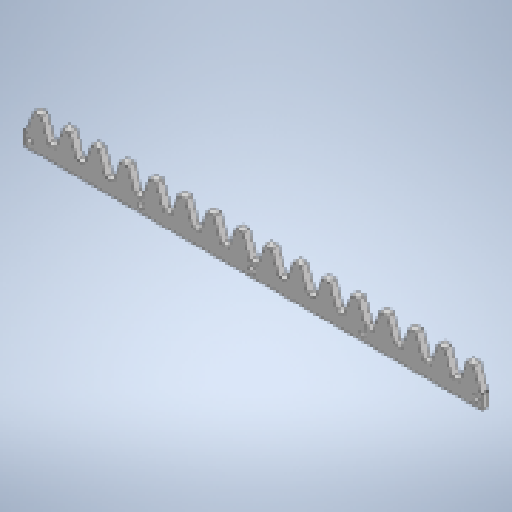
# Autodesk Inventor part: SR4-500_On
Saved by Autodesk Inventor 2024 (Build 280153000, 153)
## iProperties
Created: 2024-06-08
Part Number: SR4-500_On
Material: Generic
Catalog Web Link: www.cadenas.de
Description: Racks (SR)-
Vendor: KHK
Document SubType Name: Modeling
Designer: psAdmin
Manufacturer: KHK
Mass: 817.7 g
Surface Area: 1047.63 cm^2
Volume: 817.7 cm^3
Density: 1 g/cm^3
Appearance: PSOLRGB-175-175-175
Category: PARTsolutions
Company: KHK
PSOL_IDENT_0: {$CADENAS_DATA/23d-libs/khk/racks/racks_sr.prj},167 {VTYP=3D},{NB=SR4-500_On},{LINA=SR4-500},{NN=Rac
PSOL_IDENT_1: ks (SR)},{DATE=12.04.2024 02:30:43},{GEOMDATE=26.02.2019 12:12:45},{VERSION=},{LINEID=330},{WBVAR=TO
PSOL_IDENT_2: OTH},{WBNUMERIC=}  {NB=SR4-500_On},{LINA=SR4-500},{KT=DUMMY},{CN=SR4-500},{M=4.0},{A=505},{B=40},{C=
PSOL_IDENT_3: 45.0},{D=41.0},{ENT=39},{S=R1},{WMF=r1004},{TOOTH=On}
NB: SR4-500_On
NN: Racks (SR)
NBSYN: $CN._$TOOTH.
LINA: SR4-500
CATALOG: KHK
CN: SR4-500
M: 4
A: 505
B: 40
C: 45
D: 41
ENT: 39
S: R1
TOOTH: On
SUPPLIER: KHK
ARTICLENO: SR4-500_On
BOMINFO: SR4-500
CREATOR: CADENAS GmbH
Title: SR4-500
Author: Cadenas PARTsolutions
Autodesk Inventor part; units mm, degrees
ref_plane "YZ Plane" through (0, 0, 0) normal (1, 0, 0) x (0, 1, 0)
ref_plane "XZ Plane" through (0, 0, 0) normal (0, 1, 0) x (-1, 0, 0)
ref_plane "XY Plane" through (0, 0, 0) normal (0, 0, 1) x (1, 0, 0)
sketch "Sketch_4" plane through (0, 0, 0) normal (0, 0, 1) x (1, 0, 0)
  line L0 (0, 45) -> (0, 0)
  line L1 (0, 0) -> (505, 0)
  line L2 (505, 0) -> (505, 45)
  line L3 (505, 45) -> (0, 45)
  constraints: 8 end point
extrude "Extrusion1" add sketch "Sketch_4" along normal mid plane 40
sketch "Sketch_5" plane through (0, 0, 0) normal (0, 0, 1) x (1, 0, 0)
  line L0 (-4.714, 45) -> (-1.57, 36)
  line L1 (-1.57, 36) -> (1.57, 36)
  line L2 (1.57, 36) -> (4.714, 45)
  line L3 (4.714, 45) -> (-4.714, 45)
  constraints: 8 end point
extrude "Extrusion2" cut sketch "Sketch_5" along normal mid plane 40
pattern_linear "Rectangular Pattern1" count 42 spacing 12.56636 along (1, 0, 0) of "Extrusion2"
sketch "スケッチ3" plane through (0, 0, 20) normal (0, 0, 1) x (1, 0, 0)
  line L0 (505, 38.220229) -> (504.2244, 36)
  line L1 (504.2244, 36) -> (501.0844, 36)
  line L2 (501.0844, 36) -> (497.9404, 45)
  line L3 (497.9404, 45) -> (494.80204, 45)
  line L4 (494.80204, 45) -> (491.65804, 36)
  line L5 (491.65804, 36) -> (488.51804, 36)
  line L6 (488.51804, 36) -> (485.37404, 45)
  line L7 (485.37404, 45) -> (482.23568, 45)
  line L8 (482.23568, 45) -> (479.09168, 36)
  line L9 (479.09168, 36) -> (475.95168, 36)
  line L10 (475.95168, 36) -> (472.80768, 45)
  line L11 (472.80768, 45) -> (469.66932, 45)
  line L12 (469.66932, 45) -> (466.52532, 36)
  line L13 (466.52532, 36) -> (463.38532, 36)
  line L14 (463.38532, 36) -> (460.24132, 45)
  line L15 (460.24132, 45) -> (457.10296, 45)
  line L16 (457.10296, 45) -> (453.95896, 36)
  line L17 (453.95896, 36) -> (450.81896, 36)
  line L18 (450.81896, 36) -> (447.67496, 45)
  line L19 (447.67496, 45) -> (444.5366, 45)
  line L20 (444.5366, 45) -> (441.3926, 36)
  line L21 (441.3926, 36) -> (438.2526, 36)
  line L22 (438.2526, 36) -> (435.1086, 45)
  line L23 (435.1086, 45) -> (431.97024, 45)
  line L24 (431.97024, 45) -> (428.82624, 36)
  line L25 (428.82624, 36) -> (425.68624, 36)
  line L26 (425.68624, 36) -> (422.54224, 45)
  line L27 (422.54224, 45) -> (419.40388, 45)
  line L28 (419.40388, 45) -> (416.25988, 36)
  line L29 (416.25988, 36) -> (413.11988, 36)
  line L30 (413.11988, 36) -> (409.97588, 45)
  line L31 (409.97588, 45) -> (406.83752, 45)
  line L32 (406.83752, 45) -> (403.69352, 36)
  line L33 (403.69352, 36) -> (400.55352, 36)
  line L34 (400.55352, 36) -> (397.40952, 45)
  line L35 (397.40952, 45) -> (394.27116, 45)
  line L36 (394.27116, 45) -> (391.12716, 36)
  line L37 (391.12716, 36) -> (387.98716, 36)
  line L38 (387.98716, 36) -> (384.84316, 45)
  line L39 (384.84316, 45) -> (381.7048, 45)
  line L40 (381.7048, 45) -> (378.5608, 36)
  line L41 (378.5608, 36) -> (375.4208, 36)
  line L42 (375.4208, 36) -> (372.2768, 45)
  line L43 (372.2768, 45) -> (369.13844, 45)
  line L44 (369.13844, 45) -> (365.99444, 36)
  line L45 (365.99444, 36) -> (362.85444, 36)
  line L46 (362.85444, 36) -> (359.71044, 45)
  line L47 (359.71044, 45) -> (356.57208, 45)
  line L48 (356.57208, 45) -> (353.42808, 36)
  line L49 (353.42808, 36) -> (350.28808, 36)
  line L50 (350.28808, 36) -> (347.14408, 45)
  line L51 (347.14408, 45) -> (344.00572, 45)
  line L52 (344.00572, 45) -> (340.86172, 36)
  line L53 (340.86172, 36) -> (337.72172, 36)
  line L54 (337.72172, 36) -> (334.57772, 45)
  line L55 (334.57772, 45) -> (331.43936, 45)
  line L56 (331.43936, 45) -> (328.29536, 36)
  line L57 (328.29536, 36) -> (325.15536, 36)
  line L58 (325.15536, 36) -> (322.01136, 45)
  line L59 (322.01136, 45) -> (318.873, 45)
  line L60 (318.873, 45) -> (315.729, 36)
  line L61 (315.729, 36) -> (312.589, 36)
  line L62 (312.589, 36) -> (309.445, 45)
  line L63 (309.445, 45) -> (306.30664, 45)
  line L64 (306.30664, 45) -> (303.16264, 36)
  line L65 (303.16264, 36) -> (300.02264, 36)
  line L66 (300.02264, 36) -> (296.87864, 45)
  line L67 (296.87864, 45) -> (293.74028, 45)
  line L68 (293.74028, 45) -> (290.59628, 36)
  line L69 (290.59628, 36) -> (287.45628, 36)
  line L70 (287.45628, 36) -> (284.31228, 45)
  line L71 (284.31228, 45) -> (281.17392, 45)
  line L72 (281.17392, 45) -> (278.02992, 36)
  line L73 (278.02992, 36) -> (274.88992, 36)
  line L74 (274.88992, 36) -> (271.74592, 45)
  line L75 (271.74592, 45) -> (268.60756, 45)
  line L76 (268.60756, 45) -> (265.46356, 36)
  line L77 (265.46356, 36) -> (262.32356, 36)
  line L78 (262.32356, 36) -> (259.17956, 45)
  line L79 (259.17956, 45) -> (256.0412, 45)
  line L80 (256.0412, 45) -> (252.8972, 36)
  line L81 (252.8972, 36) -> (249.7572, 36)
  line L82 (249.7572, 36) -> (246.6132, 45)
  line L83 (246.6132, 45) -> (243.47484, 45)
  line L84 (243.47484, 45) -> (240.33084, 36)
  line L85 (240.33084, 36) -> (237.19084, 36)
  line L86 (237.19084, 36) -> (234.04684, 45)
  line L87 (234.04684, 45) -> (230.90848, 45)
  line L88 (230.90848, 45) -> (227.76448, 36)
  line L89 (227.76448, 36) -> (224.62448, 36)
  line L90 (224.62448, 36) -> (221.48048, 45)
  line L91 (221.48048, 45) -> (218.34212, 45)
  line L92 (218.34212, 45) -> (215.19812, 36)
  line L93 (215.19812, 36) -> (212.05812, 36)
  line L94 (212.05812, 36) -> (208.91412, 45)
  line L95 (208.91412, 45) -> (205.77576, 45)
  line L96 (205.77576, 45) -> (202.63176, 36)
  line L97 (202.63176, 36) -> (199.49176, 36)
  line L98 (199.49176, 36) -> (196.34776, 45)
  line L99 (196.34776, 45) -> (193.2094, 45)
  line L100 (193.2094, 45) -> (190.0654, 36)
  line L101 (190.0654, 36) -> (186.9254, 36)
  line L102 (186.9254, 36) -> (183.7814, 45)
  line L103 (183.7814, 45) -> (180.64304, 45)
  line L104 (180.64304, 45) -> (177.49904, 36)
  line L105 (177.49904, 36) -> (174.35904, 36)
  line L106 (174.35904, 36) -> (171.21504, 45)
  line L107 (171.21504, 45) -> (168.07668, 45)
  line L108 (168.07668, 45) -> (164.93268, 36)
  line L109 (164.93268, 36) -> (161.79268, 36)
  line L110 (161.79268, 36) -> (158.64868, 45)
  line L111 (158.64868, 45) -> (155.51032, 45)
  line L112 (155.51032, 45) -> (152.36632, 36)
  line L113 (152.36632, 36) -> (149.22632, 36)
  line L114 (149.22632, 36) -> (146.08232, 45)
  line L115 (146.08232, 45) -> (142.94396, 45)
  line L116 (142.94396, 45) -> (139.79996, 36)
  line L117 (139.79996, 36) -> (136.65996, 36)
  line L118 (136.65996, 36) -> (133.51596, 45)
  line L119 (133.51596, 45) -> (130.3776, 45)
  line L120 (130.3776, 45) -> (127.2336, 36)
  line L121 (127.2336, 36) -> (124.0936, 36)
  line L122 (124.0936, 36) -> (120.9496, 45)
  line L123 (120.9496, 45) -> (117.81124, 45)
  line L124 (117.81124, 45) -> (114.66724, 36)
  line L125 (114.66724, 36) -> (111.52724, 36)
  line L126 (111.52724, 36) -> (108.38324, 45)
  line L127 (108.38324, 45) -> (105.24488, 45)
  line L128 (105.24488, 45) -> (102.10088, 36)
  line L129 (102.10088, 36) -> (98.96088, 36)
  line L130 (98.96088, 36) -> (95.81688, 45)
  line L131 (95.81688, 45) -> (92.67852, 45)
  line L132 (92.67852, 45) -> (89.53452, 36)
  line L133 (89.53452, 36) -> (86.39452, 36)
  line L134 (86.39452, 36) -> (83.25052, 45)
  line L135 (83.25052, 45) -> (80.11216, 45)
  line L136 (80.11216, 45) -> (76.96816, 36)
  line L137 (76.96816, 36) -> (73.82816, 36)
  line L138 (73.82816, 36) -> (70.68416, 45)
  line L139 (70.68416, 45) -> (67.5458, 45)
  line L140 (67.5458, 45) -> (64.4018, 36)
  line L141 (64.4018, 36) -> (61.2618, 36)
  line L142 (61.2618, 36) -> (58.1178, 45)
  line L143 (58.1178, 45) -> (54.97944, 45)
  line L144 (54.97944, 45) -> (51.83544, 36)
  line L145 (51.83544, 36) -> (48.69544, 36)
  line L146 (48.69544, 36) -> (45.55144, 45)
  line L147 (45.55144, 45) -> (42.41308, 45)
  line L148 (42.41308, 45) -> (39.26908, 36)
  line L149 (39.26908, 36) -> (36.12908, 36)
  line L150 (36.12908, 36) -> (32.98508, 45)
  line L151 (32.98508, 45) -> (29.84672, 45)
  line L152 (29.84672, 45) -> (26.70272, 36)
  line L153 (26.70272, 36) -> (23.56272, 36)
  line L154 (23.56272, 36) -> (20.41872, 45)
  line L155 (20.41872, 45) -> (17.28036, 45)
  line L156 (17.28036, 45) -> (14.13636, 36)
  line L157 (14.13636, 36) -> (10.99636, 36)
  line L158 (10.99636, 36) -> (7.85236, 45)
  line L159 (7.85236, 45) -> (4.714, 45)
  line L160 (4.714, 45) -> (1.57, 36)
  line L161 (1.57, 36) -> (0, 36)
  line L162 (0, 36) -> (0, 0)
  line L163 (0, 0) -> (505, 0)
  line L164 (505, 0) -> (505, 38.220229)
  line L165 (200, 0) -> (200, 45)
  point P0 (0, 18)
  point P1 (200, 36)
  dimension "d10" = 200
  constraints: 2 end point, 1 horizontal alignment, 1 midpoint, 1 point on line, 1 vertical
  measures "d10" distance from line of point (0, 18) L165
extrude "押し出し3" cut sketch "スケッチ3" against normal through all contours L164 L163 L165 L97 L96 L95 L94 L93 L92 L91 L90 L89 L88 L87 L86 L85 L84 L83 L82 L81 L80 L79 L78 L77 L76 L75 L74 L73 L72 L71 L70 L69 L68 L67 L66 L65 L64 L63 L62 L61 L60 L59 L58 L57 L56 L55 L54 L53 L52 L51 L50 L49 L48 L47 L46 L45 L44 L43 L42 L41 L40 L39 L38 L37 L36 L35 L34 L33 L32 L31 L30 L29 L28 L27 L26 L25 L24 L23 L22 L21 L20 L19 L18 L17 L16 L15 L14 L13 L12 L11 L10 L9 L8 L7 L6 L5 L4 L3 L2 L1 L0
sketch "スケッチ4" plane through (0, 0, 20) normal (0, 0, 1) x (1, 0, 0)
  line L0 (200, 0) -> (200, 36)
  line L1 (200, 36) -> (199.49176, 36)
  line L2 (199.49176, 36) -> (196.34776, 45)
  line L3 (196.34776, 45) -> (193.2094, 45)
  line L4 (193.2094, 45) -> (190.0654, 36)
  line L5 (190.0654, 36) -> (186.9254, 36)
  line L6 (186.9254, 36) -> (183.7814, 45)
  line L7 (183.7814, 45) -> (180.64304, 45)
  line L8 (180.64304, 45) -> (177.49904, 36)
  line L9 (177.49904, 36) -> (174.35904, 36)
  line L10 (174.35904, 36) -> (171.21504, 45)
  line L11 (171.21504, 45) -> (168.07668, 45)
  line L12 (168.07668, 45) -> (164.93268, 36)
  line L13 (164.93268, 36) -> (161.79268, 36)
  line L14 (161.79268, 36) -> (158.64868, 45)
  line L15 (158.64868, 45) -> (155.51032, 45)
  line L16 (155.51032, 45) -> (152.36632, 36)
  line L17 (152.36632, 36) -> (149.22632, 36)
  line L18 (149.22632, 36) -> (146.08232, 45)
  line L19 (146.08232, 45) -> (142.94396, 45)
  line L20 (142.94396, 45) -> (139.79996, 36)
  line L21 (139.79996, 36) -> (136.65996, 36)
  line L22 (136.65996, 36) -> (133.51596, 45)
  line L23 (133.51596, 45) -> (130.3776, 45)
  line L24 (130.3776, 45) -> (127.2336, 36)
  line L25 (127.2336, 36) -> (124.0936, 36)
  line L26 (124.0936, 36) -> (120.9496, 45)
  line L27 (120.9496, 45) -> (117.81124, 45)
  line L28 (117.81124, 45) -> (114.66724, 36)
  line L29 (114.66724, 36) -> (111.52724, 36)
  line L30 (111.52724, 36) -> (108.38324, 45)
  line L31 (108.38324, 45) -> (105.24488, 45)
  line L32 (105.24488, 45) -> (102.10088, 36)
  line L33 (102.10088, 36) -> (98.96088, 36)
  line L34 (98.96088, 36) -> (95.81688, 45)
  line L35 (95.81688, 45) -> (92.67852, 45)
  line L36 (92.67852, 45) -> (89.53452, 36)
  line L37 (89.53452, 36) -> (86.39452, 36)
  line L38 (86.39452, 36) -> (83.25052, 45)
  line L39 (83.25052, 45) -> (80.11216, 45)
  line L40 (80.11216, 45) -> (76.96816, 36)
  line L41 (76.96816, 36) -> (73.82816, 36)
  line L42 (73.82816, 36) -> (70.68416, 45)
  line L43 (70.68416, 45) -> (67.5458, 45)
  line L44 (67.5458, 45) -> (64.4018, 36)
  line L45 (64.4018, 36) -> (61.2618, 36)
  line L46 (61.2618, 36) -> (58.1178, 45)
  line L47 (58.1178, 45) -> (54.97944, 45)
  line L48 (54.97944, 45) -> (51.83544, 36)
  line L49 (51.83544, 36) -> (48.69544, 36)
  line L50 (48.69544, 36) -> (45.55144, 45)
  line L51 (45.55144, 45) -> (42.41308, 45)
  line L52 (42.41308, 45) -> (39.26908, 36)
  line L53 (39.26908, 36) -> (36.12908, 36)
  line L54 (36.12908, 36) -> (32.98508, 45)
  line L55 (32.98508, 45) -> (29.84672, 45)
  line L56 (29.84672, 45) -> (26.70272, 36)
  line L57 (26.70272, 36) -> (23.56272, 36)
  line L58 (23.56272, 36) -> (20.41872, 45)
  line L59 (20.41872, 45) -> (17.28036, 45)
  line L60 (17.28036, 45) -> (14.13636, 36)
  line L61 (14.13636, 36) -> (10.99636, 36)
  line L62 (10.99636, 36) -> (7.85236, 45)
  line L63 (7.85236, 45) -> (4.714, 45)
  line L64 (4.714, 45) -> (1.57, 36)
  line L65 (1.57, 36) -> (0, 36)
  line L66 (0, 36) -> (0, 0)
  line L67 (0, 0) -> (200, 0)
extrude "押し出し4" cut sketch "スケッチ4" against normal blind 37
sketch "スケッチ5" plane through (0, 0, -17) normal (0, 0, 1) x (1, 0, 0)
  line L0 (0, 0) -> (0, 36)
  line L1 (0, 27) -> (200, 27)
  line L2 (200, 36) -> (200, 0)
  line L3 (155.51032, 45) -> (158.64868, 45)
  circle A0 centre (4.5, 31.5) radius 4.5 construction
  line L4 (0, 36) -> (1.57, 36)
  circle A1 centre (4.5, 31.5) radius 1.3
  line L5 (100, 27) -> (100, 0) construction
  circle A2 centre (100, 31.5) radius 1.3
  circle A3 centre (195.5, 31.5) radius 1.3
  line L6 (4.5, 31.5) -> (100, 31.5) construction
  circle A4 centre (52.25, 31.5) radius 1.3
  circle A5 centre (147.75, 31.5) radius 1.3
  line L7 (200, 0) -> (0, 0)
  point P0 (157.0795, 45)
  dimension "d15" = 18
  dimension "d16" = 2.6
  dimension "d17" = 2.6
  dimension "d18" = 2.6
  constraints: 6 centre point, 6 end point, 3 midpoint, 3 tangent, 2 horizontal, 2 point on line, 2 symmetric about line, 1 coincident, 1 horizontal alignment, 1 vertical, 1 vertical alignment, 2 other
  measures "d15" distance from line of point (157.079, 45) L1
  measures "d16" diameter of A1
  measures "d17" diameter of A2
  measures "d18" diameter of A4
extrude "押し出し5" cut sketch "スケッチ5" against normal through all
body "Solid1"
